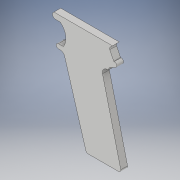
# Autodesk Inventor part: remote_housing_top
Saved by Autodesk Inventor 2019.4 (Build 234330000, 330)
## iProperties
Created: 2019-10-02
Part Number: remote_housing_top
Material: Generic
Document SubType Name: Modeling
Designer: nLaptop
Density: 1 g/cm^3
Appearance: Default
Author: nLaptop
Autodesk Inventor part; units mm, degrees
ref_plane "YZ Plane" through (0, 0, 0) normal (1, 0, 0) x (0, 1, 0)
ref_plane "XZ Plane" through (0, 0, 0) normal (0, 1, 0) x (-1, 0, 0)
ref_plane "XY Plane" through (0, 0, 0) normal (0, 0, 1) x (1, 0, 0)
sketch "Sketch1" plane through (0, 0, 0) normal (0, 0, 1) x (1, 0, 0)
  line L0 (27.1259, 158.6213) -> (27.9311, 158.6213)
  line L1 (29.361, 152.6115) -> (22.335, 149.0674)
  arc A0 (29.361, 152.6115) -> (27.9311, 158.6213) centre (27.9311, 155.4463) ccw
  arc A1 (22.335, 149.0674) -> (20.6334, 145.7092) centre (23.7649, 146.2326) ccw
  line L2 (22.0403, 169.1855) -> (27.1259, 158.6213)
  arc A2 (22.634, 172.5449) -> (22.0403, 169.1855) centre (24.6722, 170.4525) ccw
  line L3 (-6.41, 36.887) -> (33.4699, 36.887)
  line L4 (-6.41, 36.887) -> (-6.4982, 36.887)
  arc A3 (-9.358, 39.2132) -> (-6.4982, 36.887) centre (-6.4982, 39.808) ccw
  arc A4 (33.4699, 36.887) -> (36.359, 40.2384) centre (33.4699, 39.808) ccw
  line L5 (-9.358, 39.2132) -> (-37.1084, 132.0559)
  line L6 (36.359, 40.2384) -> (12.4496, 137.1498)
  line L7 (17.0937, 144.836) -> (20.6334, 145.7092)
  arc A5 (17.0937, 144.836) -> (12.4496, 137.1498) centre (18.6147, 138.6708) ccw
  arc A6 (-37.1084, 132.0559) -> (-43.1527, 136.5873) centre (-43.1924, 130.2374) ccw
  line L8 (-43.1527, 136.5873) -> (-45.1745, 136.5873)
  arc A7 (-45.1745, 142.4293) -> (-45.1745, 136.5873) centre (-45.1745, 139.5083) ccw
  line L9 (-45.1745, 142.4293) -> (-38.8245, 142.4293)
  line L10 (-44.129, 168.0864) -> (-49.28, 168.0864)
  arc A8 (-38.8245, 142.4293) -> (-42.3029, 167.4452) centre (-53.7957, 153.0974) ccw
  arc A9 (-42.3029, 167.4452) -> (-44.129, 168.0864) centre (-44.129, 165.1654) ccw
  line L11 (-51.1648, 175.285) -> (25.447, 175.285)
  line L12 (22.634, 172.5449) -> (25.447, 175.285)
  arc A10 (-51.1648, 175.285) -> (-49.28, 168.0864) centre (-49.28, 171.9325) ccw
  point P0 (-38.454, 136.5579)
  point P1 (-43.1527, 168.0864)
  dimension "d10" = 3.175
  dimension "d21" = 2.921
  dimension "d23" = 2.921
  dimension "d24" = 101.6
  dimension "d27" = 6.35
  dimension "d29" = 6.35
  dimension "d30" = 2.921
  constraints: 26 end point, 23 point on circle, 13 tangent, 11 centre point, 6 horizontal, 2 equal radius, 2 point on line, 1 perpendicular
  measures "d10" radius of A0
  measures "d21" radius of A2
  measures "d23" radius of A3
  measures "d24" distance of L5.start point (-38.454, 136.558)
  measures "d27" radius of A6
  measures "d29" distance of L9.start L9.end
  measures "d30" radius of A9
extrude "Extrusion1" add sketch "Sketch1" along normal blind 8.89
shell "Shell3" thickness 2.54 removed faces 1 at (-11.339, 102.8063, 0)
body "Solid1"
